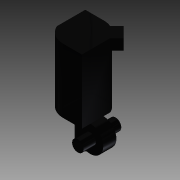
# Autodesk Inventor part: Motor_500RPM
Saved by Autodesk Inventor 2015 (Build 190159000, 159)
## iProperties
Created: 2015-07-12
Part Number: Motor_500RPM
Material: Aluminum 6061
Document SubType Name: Modeling
Designer: k
Density: 2.7 g/cm^3
Appearance: Aluminum - Flat
Author: k
Autodesk Inventor part; units mm, degrees
ref_plane "YZ Plane" through (0, 0, 0) normal (1, 0, 0) x (0, 1, 0)
ref_plane "XZ Plane" through (0, 0, 0) normal (0, 1, 0) x (-1, 0, 0)
ref_plane "XY Plane" through (0, 0, 0) normal (0, 0, 1) x (1, 0, 0)
sketch "Sketch1" plane through (0, 0, 0) normal (0, 1, 0) x (-1, 0, 0)
  line L0 (-25.8445, -28.2321) -> (25.8445, -28.2321) construction
  line L1 (25.8445, -28.2321) -> (25.8445, 28.2321) construction
  line L2 (25.8445, 28.2321) -> (-25.8445, 28.2321) construction
  line L3 (-25.8445, 28.2321) -> (-25.8445, -28.2321) construction
  line L4 (-25.8445, -28.2321) -> (25.8445, 28.2321) construction
  line L5 (25.8445, -28.2321) -> (-25.8445, 28.2321) construction
  circle A0 centre (0, 0) radius 28.2321 construction
  arc A1 (-25.8445, -11.3628) -> (0, -28.2321) centre (0, 0) ccw
  arc A2 (25.8445, 11.3628) -> (0, 28.2321) centre (0, 0) ccw
  line L6 (25.8445, 11.3628) -> (25.8445, -28.2321)
  line L7 (25.8445, -28.2321) -> (0, -28.2321)
  line L8 (-25.8445, -11.3628) -> (-25.8445, 28.2321)
  line L9 (-25.8445, 28.2321) -> (0, 28.2321)
  dimension "d2" = 51.689
  dimension "d3" = 56.4642
  constraints: 20 end point, 8 point on circle, 3 centre point, 3 midpoint, 2 concentric, 2 parallel, 2 perpendicular, 2 point on line, 2 tangent, 1 collinear, 1 horizontal, 1 vertical
  measures "d2" distance of L2.end L1.end
  measures "d3" distance of L1.end L0.end
extrude "Extrusion1" add sketch "Sketch1" along normal blind 89.4842
sketch "Sketch2" plane through (0, 0, 0) normal (0, -1, 0) x (1, 0, 0)
  circle A0 centre (0, 0) radius 8.89
  dimension "d6" = 17.78
  constraints: 1 centre point
  measures "d6" diameter of A0
extrude "Extrusion2" add sketch "Sketch2" along normal blind 48.26
sketch "Sketch3" plane through (0, 0, 0) normal (0, 0, 1) x (1, 0, 0)
  line L0 (-8.89, -48.26) -> (8.89, -48.26) projected
  line L1 (8.89, 0) -> (-8.89, 0) projected
  line L2 (0, -48.26) -> (0, -25.4) construction
  line L3 (0, -25.4) -> (18.288, -25.4) construction
  circle A0 centre (18.288, -25.4) radius 18.288
  dimension "d9" = 22.86
  dimension "d10" = 18.288
  constraints: 4 end point, 1 coincident, 1 horizontal, 1 horizontal alignment, 1 midpoint, 1 vertical, 2 other
  measures "d9" distance of L2.start L2.end
  measures "d10" distance of L2.end L3.end
extrude "Extrusion3" add sketch "Sketch3" along normal blind 9.144 and the other way blind 9.144
sketch "Sketch4" plane through (18.288, -25.4, 9.144) normal (0, 0, 1) x (1, 0, 0)
  circle A0 centre (0, 0) radius 8.001
  dimension "d15" = 16.002
  constraints: 1 centre point
  measures "d15" diameter of A0
extrude "Extrusion4" add sketch "Sketch4" along normal blind 17.145
mirror "Mirror1" about plane through (0, 0, 0) normal (0, 0, 1) of "Extrusion4"
sketch "Sketch5" plane through (0, 89.4842, 0) normal (0, 1, 0) x (1, 0, 0)
  arc A0 (25.8445, 11.3628) -> (0, 28.2321) centre (0, 0) ccw construction
  line L0 (25.8445, -28.2321) -> (25.8445, 11.3628) construction
  line L1 (25.8445, 11.3628) -> (35.184, 20.7023)
  line L2 (25.8445, 11.3628) -> (39.0525, 11.3628) construction
  line L3 (35.184, 20.7023) -> (20.4563, 35.4299)
  line L4 (20.4563, 35.4299) -> (11.0193, 25.9928)
  arc A1 (25.8445, 11.3628) -> (11.0193, 25.9928) centre (0, 0) ccw
  dimension "d18" = 13.208
  dimension "d19" = 45
  dimension "d20" = 20.828
  constraints: 8 end point, 3 point on circle, 2 perpendicular, 1 centre point, 1 concentric, 1 equal length, 1 horizontal
  measures "d18" distance of L0.end L1.end
  measures "d19" angle of L2 L1
  measures "d20" distance of L1.end L3.end
extrude "Extrusion5" add sketch "Sketch5" against normal blind 15.24
body "Solid1"
